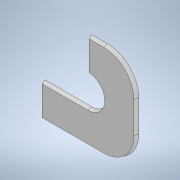
# Autodesk Inventor part: hook
Saved by Autodesk Inventor 2020 (Build 240168000, 168)
## iProperties
Created: 2020-01-24
Part Number: hook
Material: Generic
Document SubType Name: Modeling
Designer: 1sfkeith
Density: 1 g/cm^3
Appearance: Default
Author: 1sfkeith
Autodesk Inventor part; units mm, degrees
ref_plane "YZ Plane" through (0, 0, 0) normal (1, 0, 0) x (0, 1, 0)
ref_plane "XZ Plane" through (0, 0, 0) normal (0, 1, 0) x (-1, 0, 0)
ref_plane "XY Plane" through (0, 0, 0) normal (0, 0, 1) x (1, 0, 0)
sketch "Sketch1" plane through (0, 0, 0) normal (0, 0, 1) x (1, 0, 0)
  line L0 (198.6992, 341.4095) -> (224.0992, 341.4095)
  line L1 (274.8992, 290.6095) -> (274.8992, 239.8095)
  line L2 (224.0992, 189.0095) -> (122.4992, 189.0095)
  line L3 (198.4116, 290.6095) -> (198.6992, 290.6095)
  line L4 (224.0992, 265.2095) -> (224.0992, 265.2095)
  line L5 (198.6992, 239.8095) -> (122.4992, 239.8095)
  line L6 (198.6992, 341.4095) -> (198.6992, 290.6095)
  line L7 (122.4992, 239.8095) -> (122.4992, 189.0095)
  arc A0 (224.0992, 265.2095) -> (198.6992, 290.6095) centre (198.6992, 265.2095) ccw
  arc A1 (198.6992, 239.8095) -> (224.0992, 265.2095) centre (198.6992, 265.2095) ccw
  arc A2 (274.8992, 290.6095) -> (224.0992, 341.4095) centre (224.0992, 290.6095) ccw
  arc A3 (224.0992, 189.0095) -> (274.8992, 239.8095) centre (224.0992, 239.8095) ccw
  circle A4 centre (143.7935, 214.4095) radius 12.7
  point P0 (0, 0)
  point P1 (274.8992, 341.4095)
  point P2 (274.8992, 189.0095)
  point P3 (274.8992, 265.2095)
  dimension "d0" = 50.8
  dimension "d1" = 50.8
  dimension "d2" = 50.8
  dimension "d3" = 50.8
  dimension "d6" = 152.4
  dimension "d7" = 25.4
  dimension "d8" = 25.4
  dimension "d9" = 50.8
  dimension "d12" = 25.4
  constraints: 16 end point, 8 point on circle, 8 tangent, 5 centre point, 5 point on line, 4 horizontal, 1 equal radius, 1 vertical
  measures "d0" distance between parallel lines of L5 L3
  measures "d1" distance between parallel lines of L3 L0
  measures "d2" distance between parallel lines of L2 L5
  measures "d3" distance between parallel lines of L1 L4
  measures "d6" distance of point (274.899, 189.01) L2.end
  measures "d7" radius of A0
  measures "d8" radius of A1
  measures "d9" radius of A2
  measures "d12" diameter of A4
extrude "Extrusion1" add sketch "Sketch1" along normal blind 6.35 draft -15 contours L0 A2 L1 A3 L2 L7 L5 A1 A0 L6 | A4
body "Solid1"
